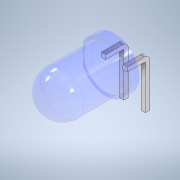
# Autodesk Inventor part: IR_TSAL6400
Saved by Autodesk Inventor 2021 (Build 250183000, 183)
## iProperties
Created: 2020-03-26
Part Number: IR_TSAL6400
Material: Generic
Document SubType Name: Modeling
Designer: ermoz
Density: 1 g/cm^3
Appearance: Default
Mass: 0.191085 g
Surface Area: 4.5397 cm^2
Volume: 0.191085 cm^3
Author: ermoz
Autodesk Inventor part; units mm, degrees
ref_plane "YZ Plane" through (0, 0, 0) normal (1, 0, 0) x (0, 1, 0)
ref_plane "XZ Plane" through (0, 0, 0) normal (0, 1, 0) x (-1, 0, 0)
ref_plane "XY Plane" through (0, 0, 0) normal (0, 0, 1) x (1, 0, 0)
sketch "Sketch1" plane through (0, 0, 0) normal (1, 0, 0) x (0, 1, 0)
  line L0 (0, 0) -> (2.5, 0)
  line L1 (2.5, 0) -> (2.5, 8.5)
  line L2 (2.5, 8.5) -> (0, 8.5)
  line L3 (0, 8.5) -> (0, 0)
  line L4 (2.5, 0) -> (2.875, 0)
  line L5 (2.875, 0) -> (2.875, 1)
  line L6 (2.875, 1) -> (2.5, 1)
  line L7 (2.5, 1) -> (2.5, 0)
  arc A0 (0, 3.5) -> (0, 8.5) centre (0, 6) ccw
  point P0 (2.5, 6)
  dimension "d0" = 2.5
  dimension "d1" = 8.5
  dimension "d2" = 0.375
  dimension "d3" = 1
  constraints: 16 end point, 4 parallel, 2 horizontal, 2 perpendicular, 2 point on circle, 1 centre point, 1 point on line, 1 tangent
  measures "d0" distance of L2.end L1.end
  measures "d1" distance of L1.end L0.end
  measures "d2" distance of L6.end L5.end
  measures "d3" distance of L5.end L4.end
revolve "Revolution1" add sketch "Sketch1" angle 360 about axis through (0, 0, 8.5) along (0, 0, -1) contours L3 A0 L1 L0 | L1 L6 L5 L4 | L3 A0
sketch "Sketch2" plane through (0, 0, 0) normal (0, 0, -1) x (-1, 0, 0)
  circle A0 centre (0, 0) radius 2.875 projected
  line L0 (0, 0) -> (2.589, 0)
  line L1 (2.589, 0) -> (2.589, 1.25)
  line L2 (2.589, 1.25) -> (0, 1.25)
  line L3 (0, 1.25) -> (0, 0)
  line L4 (0, 0) -> (2.589, 0)
  line L5 (2.589, 0) -> (2.589, -1.25)
  line L6 (2.589, -1.25) -> (0, -1.25)
  line L7 (0, -1.25) -> (0, 0)
  arc A1 (2.589, -1.25) -> (2.589, 1.25) centre (0, 0) ccw
  dimension "d5" = 1.25
  dimension "d6" = 1.25
  constraints: 16 end point, 4 parallel, 2 horizontal, 2 perpendicular, 2 point on circle, 1 centre point, 1 point on line, 3 other
  measures "d5" distance of L1.end L0.end
  measures "d6" distance of L4.end L5.end
extrude "Extrusion1" cut sketch "Sketch2" against normal blind 10 contours A0 L5 L1
sketch "Sketch3" plane through (0, 0, 0) normal (0, 0, -1) x (-1, 0, 0)
  line L0 (0, 0) -> (-1.5, 0)
  line L1 (-1.5, 0) -> (-1.25, 0)
  line L2 (-1, -0.25) -> (-1.5, -0.25)
  line L3 (-1.5, -0.25) -> (-1.5, 0.25)
  line L4 (-1.5, 0.25) -> (-1, 0.25)
  line L5 (-1, 0.25) -> (-1, -0.25)
  line L6 (-1, -0.25) -> (-1.5, 0.25) construction
  line L7 (-1.5, -0.25) -> (-1, 0.25) construction
  line L8 (0, 0) -> (1.25, 0)
  line L9 (1.5, -0.25) -> (1, -0.25)
  line L10 (1, -0.25) -> (1, 0.25)
  line L11 (1, 0.25) -> (1.5, 0.25)
  line L12 (1.5, 0.25) -> (1.5, -0.25)
  line L13 (1.5, -0.25) -> (1, 0.25) construction
  line L14 (1, -0.25) -> (1.5, 0.25) construction
  dimension "d9" = 1.5
  dimension "d10" = 0.25
  dimension "d11" = 0.5
  dimension "d12" = 1.25
  dimension "d13" = 0.5
  dimension "d14" = 0.5
  constraints: 30 end point, 4 horizontal, 4 midpoint, 4 parallel, 2 perpendicular, 1 point on line
  measures "d9" distance of L0.start L0.end
  measures "d10" distance of L0.end L1.end
  measures "d11" distance of L2.end L3.end
  measures "d12" distance of L0.start L8.end
  measures "d13" distance of L10.end L11.end
  measures "d14" distance of L9.end L10.end
extrude "Extrusion2" add sketch "Sketch3" along normal blind 2 separate body
sketch "Sketch5" plane through (1.5, -0.25, 0) normal (1, 0, 0) x (0, 0, -1)
  line L0 (0, 0) -> (2, 0) projected
  line L1 (2, 0) -> (2, -0.1)
  line L2 (2, -0.1) -> (2.1, -0.1)
  arc A0 (2.1, -0.1) -> (2, 0) centre (2, -0.1) ccw
  line L3 (2.1, -0.1) -> (2.6, -0.1)
  line L4 (0, 0.5) -> (2, 0.5) projected
  arc A1 (2.6, -0.1) -> (2, 0.5) centre (2, -0.1) ccw
  line L5 (2.1, -0.1) -> (2.6, -0.1)
  line L6 (2.6, -0.1) -> (2.6, -5.1)
  line L7 (2.6, -5.1) -> (2.1, -5.1)
  line L8 (2.1, -5.1) -> (2.1, -0.1)
  line L9 (0, 0.5) -> (2, 0.5) projected
  line L10 (2, 0.5) -> (2, 0)
  point P0 (0, 0.25)
  dimension "d20" = 0.1
  dimension "d21" = 0.1
  dimension "d22" = 0.1
  dimension "d23" = 0.5
  dimension "d24" = 0.6
  dimension "d25" = 5
  constraints: 16 end point, 4 point on circle, 3 perpendicular, 2 centre point, 2 horizontal, 2 parallel, 1 vertical
  measures "d20" distance of L0.end L1.end
  measures "d21" distance of L1.end L2.end
  measures "d22" radius of A0
  measures "d23" distance of L2.end L3.end
  measures "d24" radius of A1
  measures "d25" distance of L5.end L6.end
extrude "Extrusion4" add sketch "Sketch5" against normal blind 3 contours L10 A1 L3 A0 | L3 L6 L7 L8 bodies 2
extrude "Extrusion5" cut sketch "Sketch5" against normal blind 2.5 contours L10 A1 L3 A0 | L3 L6 L7 L8 bodies 2
extrude "Extrusion6" add sketch "Sketch5" against normal blind 0.5 contours L10 A1 L3 A0 | L3 L6 L7 L8 bodies 2
body "Solid1"
body "Solid2"
